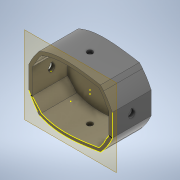
# Autodesk Inventor part: CameraHolder2
Saved by Autodesk Inventor 2021.1 (Build 251245010, 245A)
## iProperties
Created: 2023-07-02
Part Number: CameraHolder2
Material: ABS Plastic
Document SubType Name: Modeling
Designer: Drake
Density: 1.06 g/cm^3
Appearance: Smooth - White
Author: Drake
Autodesk Inventor part; units mm, degrees
sketch "Sketch1" plane through (0, 0, 0) normal (0, 0, 1) x (1, 0, 0)
  circle A0 centre (0, 0) radius 75
  line L0 (-56.0863, 49.7929) -> (-26.079, 63.6592) construction
  line L1 (-26.079, 63.6592) -> (7.2114, 60.0923) construction
  line L2 (7.2114, 60.0923) -> (53.8052, 52.2494) construction
  spline S0 degree 3 poles (-56.0863, 49.7929) (-26.079, 63.6592) (7.2114, 60.0923) (53.8052, 52.2494) knots 1 1 1 1 2 2 2 2
  line L3 (-75, 0) -> (75, 0)
  line L4 (-56.0863, -49.7929) -> (-26.079, -63.6592) construction
  line L5 (-26.079, -63.6592) -> (7.2114, -60.0923) construction
  line L6 (7.2114, -60.0923) -> (53.8052, -52.2494) construction
  spline S1 degree 3 poles (-56.0863, -49.7929) (-26.079, -63.6592) (7.2114, -60.0923) (53.8052, -52.2494) knots 1 1 1 1 2 2 2 2
  line L7 (0, 0) -> (0, 49.152)
  line L8 (-75, 0) -> (-75, 20)
  line L9 (-75, 20) -> (-75, -20)
  line L10 (0, 49.152) -> (0, -37.3687)
  line L11 (75, 20) -> (75, -20)
  arc A1 (-56.0863, 49.7929) -> (-75, 20) centre (35.1269, -29.013) ccw
  line L12 (0, 49.152) -> (0, 75)
  line L13 (0, 75) -> (0, -75.7102)
  line L14 (-75, 0) -> (75, 0)
  arc A2 (75, 20) -> (56.0863, 49.7929) centre (-35.1269, -29.013) ccw
  line L15 (-115.8608, 0) -> (95.4779, 0)
  line L16 (-56.0863, -49.7929) -> (-26.079, -63.6592) construction
  line L17 (-26.079, -63.6592) -> (7.2114, -60.0923) construction
  line L18 (7.2114, -60.0923) -> (53.8052, -52.2494) construction
  spline S2 degree 3 poles (-56.0863, -49.7929) (-26.079, -63.6592) (7.2114, -60.0923) (53.8052, -52.2494) knots 1 1 1 1 2 2 2 2
  arc A3 (-75, -20) -> (-56.0863, -49.7929) centre (35.1269, 29.013) ccw
  arc A4 (56.0863, -49.7929) -> (75, -20) centre (-35.1269, 29.013) ccw
  point P0 (0, 4.9536)
  point P1 (0, 5)
  point P2 (0.1096, -4.9988)
  point P3 (0.1096, 4.9988)
  point P4 (-59.4923, -45.6691)
  point P5 (-59.4923, 45.6691)
  point P6 (59.4923, -45.6691)
  point P7 (59.4923, 45.6691)
  dimension "d11" = 49.1519
  dimension "motorlw" = 20
  dimension "d19" = 40
  constraints: 20 end point, 13 point on circle, 11 symmetric about line, 5 centre point, 4 point on line, 3 vertical, 1 coincident, 1 collinear, 1 horizontal, 1 tangent, 12 other
  measures "d11" distance of L7.start L7.end
  measures "motorlw" distance of L3.start L8.end
  measures "d19" distance of L8.end L9.end
sketch "Sketch2" plane through (0, 0, 0) normal (1, 0, 0) x (0, 1, 0)
  point P0 (0, 0)
extrude "Extrusion1" add sketch "Sketch1" against normal mid plane 70 contours A2 A0 L3 L7 L12 S0 | A0 A2 | A2 L11 A0 | L12 L7 L3 A0 A1 S0 | L11 A4 A0 | A0 A4 S1 L13 L10 L3 | A1 A0 | A0 A4 | L10 L13 S1 A3 A0 L3 | A0 L8 A1 | A0 A3 L9 | A3 A0
sketch "Sketch3" plane through (0, 0, 35) normal (0, 0, 1) x (1, 0, 0)
  spline S0 degree 3 poles (53.8052, 52.2494) (7.2114, 60.0923) (-26.079, 63.6592) (-56.0863, 49.7929) knots 0 0 0 0 1 1 1 1
  arc A0 (-56.0863, 49.7929) -> (-56.0863, -49.7929) centre (0, 0) ccw projected
  arc A1 (53.8052, -52.2494) -> (53.8052, 52.2494) centre (0, 0) ccw projected
  spline S1 degree 3 poles (-56.0863, -49.7929) (-26.079, -63.6592) (7.2114, -60.0923) (53.8052, -52.2494) knots 0 0 0 0 1 1 1 1
  arc A2 (50.8269, -46.665) -> (50.8269, 46.665) centre (0, 0) ccw
  arc A3 (-52.4207, 44.8673) -> (-52.4207, -44.8673) centre (0, 0) ccw
  arc A4 (-59.4923, 45.6691) -> (-75, 20) centre (35.1269, -29.013) ccw projected
  line L0 (-75, 20) -> (-75, -20) projected
  arc A5 (-75, -20) -> (-59.4923, -45.6691) centre (35.1269, 29.013) ccw projected
  arc A6 (59.4923, -45.6691) -> (75, -20) centre (-35.1269, 29.013) ccw projected
  line L1 (75, -20) -> (75, 20) projected
  arc A7 (75, 20) -> (59.4923, 45.6691) centre (-35.1269, -29.013) ccw projected
  arc A8 (69, 18.7081) -> (54.7826, 41.9518) centre (-35.1269, -29.013) ccw
  line L2 (69, 18.7081) -> (69, -18.7081)
  arc A9 (54.7826, -41.9518) -> (69, -18.7081) centre (-35.1269, 29.013) ccw
  arc A10 (-54.7826, 41.9518) -> (-69, 18.7081) centre (35.1269, -29.013) ccw
  line L3 (-69, 18.7081) -> (-69, -18.7081)
  arc A11 (-69, -18.7081) -> (-54.7826, -41.9518) centre (35.1269, 29.013) ccw
  line L4 (-69, 18.7081) -> (-52.4207, 44.8673)
  line L5 (-69, 18.7081) -> (-69, -18.7081)
  line L6 (-75, -20) -> (-75, 20) projected
  line L7 (50.8269, -46.665) -> (69, -18.7081)
  line L8 (69, 18.7081) -> (50.8269, 46.665)
  line L9 (-69, 18.7081) -> (-69, -18.7081)
  line L10 (-52.4207, -44.8673) -> (-36.8956, -50.1281)
  line L11 (-69, 0) -> (-69, -18.7081)
  line L12 (-60.7667, -32.6866) -> (-69, -18.7081)
  line L13 (-69, 0) -> (-69, -26.3552)
  line L14 (-69, -26.3552) -> (-52.4207, -44.8673)
  spline S2 degree 5 poles (-52.4207, 44.8672) (-47.019, 47.2709) (-41.4169, 49.2276) (-35.6608, 50.6933) (-22.9695, 52.9234) (-10.0817, 53.3954) (-3.1266, 53.2539) (11.8982, 52.3429) (26.8335, 50.4559) (34.8446, 49.2778) (42.8405, 47.9987) (50.8269, 46.665) knots 0 0 0 0 0 0 0.282115 0.282115 0.282115 0.613647 0.613647 0.613647 1 1 1 1 1 1
  spline S3 degree 5 poles (50.8269, -46.665) (42.8405, -47.9987) (34.8446, -49.2778) (26.8335, -50.4559) (11.8982, -52.3429) (-3.1266, -53.2539) (-10.0817, -53.3954) (-22.9695, -52.9234) (-35.6608, -50.6933) (-41.4169, -49.2276) (-47.019, -47.2709) (-52.4207, -44.8672) knots 0 0 0 0 0 0 0.386353 0.386353 0.386353 0.717885 0.717885 0.717885 1 1 1 1 1 1
  point P0 (63.2794, 27.5085)
  point P1 (69, 0)
  point P2 (63.2794, -27.5085)
  point P3 (-62.9504, 28.2533)
  point P4 (-69, 0)
  point P5 (-69, 0)
  dimension "d4" = 6
  dimension "d20" = 6
  dimension "d21" = 6
  constraints: 24 end point, 14 point on circle, 6 centre point, 3 concentric, 1 collinear, 1 midpoint, 1 parallel, 1 point on line, 1 tangent, 13 other
  measures "d20" radial gap between concentric circles of A7 A8
  measures "d21" radial gap between concentric circles of A4 A10
extrude "Extrusion2" cut sketch "Sketch3" against normal blind 64 contours L7 A2 | S3 L10 A3 L4 S2 L8 A2 L7 | A2 L2 L7 | S3 L10 | A2 L8 L2 | L14 L13 A11 A3 | L8 A2 | A11 L12 A3 | L12 L3 A3 | L4 A3 | L3 L4 A3
ref_plane "Work Plane1" through (60, 0, 0) normal (1, 0, 0) x (0, 1, 0)
sketch "Sketch4" plane through (60, 0, 0) normal (1, 0, 0) x (0, 1, 0)
  arc A0 (5.25, 2.9047) -> (5.25, -2.9047) centre (0, 0) ccw
  arc A1 (5.25, -2.9047) -> (5.25, 2.9047) centre (6, 0) ccw
  dimension "motorcrescenttop" = 12
  dimension "crescent" = 6
  constraints: 5 point on circle, 2 centre point, 1 coincident
  measures "motorcrescenttop" diameter of A0
  measures "crescent" diameter of A1
extrude "Extrusion3" cut sketch "Sketch4" against normal mid plane 300
ref_plane "Work Plane2" through (0, 49.152, 0) normal (0, 1, 0) x (-1, 0, 0)
sketch "Sketch5" plane through (0, 49.152, 0) normal (0, 1, 0) x (-1, 0, 0)
  circle A0 centre (0, 0) radius 5
  dimension "d13" = 10
  constraints: 1 centre point, 1 coincident
  measures "d13" diameter of A0
mirror "Mirror1" about plane through (0, 0, 0) normal (0, 0, 1) of "Extrusion3"
ref_plane "Work Plane3" through (70, 0, 0) normal (1, 0, 0) x (0, 1, 0)
extrude "Extrusion4" cut sketch "Sketch5" against normal through all both and the other way through all
ref_plane "Work Plane4" through (0, 0, 35) normal (0, 0, 1) x (1, 0, 0)
sketch "Sketch6" plane through (0, 0, 35) normal (0, 0, 1) x (1, 0, 0)
  line L0 (-52.4207, -44.8673) -> (-69, -26.3552) projected
  arc A0 (-75, -20) -> (-59.4923, -45.6691) centre (35.1269, 29.013) ccw projected
  arc A1 (50.8269, -46.665) -> (63.2794, -27.5085) centre (0, 0) ccw projected
  arc A2 (53.8052, -52.2494) -> (59.4923, -45.6691) centre (0, 0) ccw projected
  arc A3 (59.4923, -45.6691) -> (75, -20) centre (-35.1269, 29.013) ccw projected
  line L1 (69, -18.7081) -> (63.2794, -27.5085) projected
  line L2 (-69, -26.3552) -> (-71.9458, -26.3552)
  arc A4 (-75, -20) -> (-59.4923, -45.6691) centre (35.1269, 29.013) ccw projected
  line L3 (69, -18.7081) -> (63.2794, -27.5085) projected
  line L4 (75, 20) -> (75, -20) projected
  line L5 (69, -18.7081) -> (75, -20)
  constraints: 4 end point, 1 horizontal, 1 point on circle, 2 other
equation "\"d2\" = d1"
equation "\"d1\" = 70"
body "Solid1"
